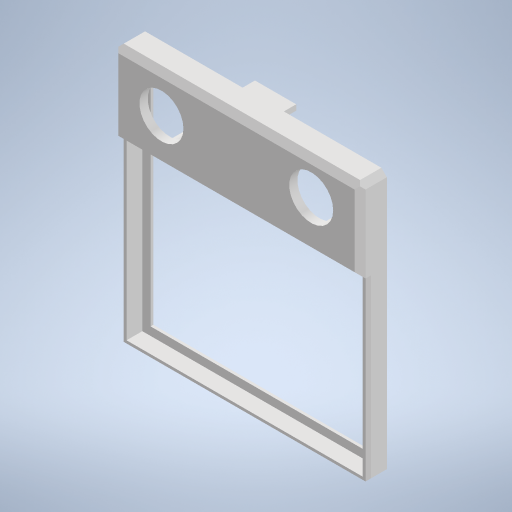
# Autodesk Inventor part: Top
Saved by Autodesk Inventor 2023.1 (Build 271208000, 208)
## iProperties
Created: 2023-03-16
Part Number: Top
Material: Generisch
Document SubType Name: Modeling
Designer: nikla
Density: 1 g/cm^3
Appearance: Vorgabe
Author: nikla
Autodesk Inventor part; units mm, degrees
ref_plane "YZ Plane" through (0, 0, 0) normal (1, 0, 0) x (0, 1, 0)
ref_plane "XZ Plane" through (0, 0, 0) normal (0, 1, 0) x (-1, 0, 0)
ref_plane "XY Plane" through (0, 0, 0) normal (0, 0, 1) x (1, 0, 0)
sketch "Skizze1" plane through (0, 0, 0) normal (0, 0, 1) x (1, 0, 0)
  line L0 (44.95, -45.95) -> (44.95, 45.95) projected
  line L1 (42.95, 47.95) -> (7.5, 47.95) projected
  line L2 (7.5, 44.95) -> (7.5, 47.95) projected
  line L3 (15, 44.95) -> (7.5, 44.95) projected
  line L4 (15, 44.95) -> (15, 42.95) projected
  line L5 (15, 42.95) -> (39.95, 42.95) projected
  line L6 (39.95, 42.95) -> (39.95, -42.95) projected
  line L7 (39.95, -42.95) -> (-39.95, -42.95) projected
  line L8 (-39.95, -42.95) -> (-39.95, 42.95) projected
  line L9 (-39.95, 42.95) -> (-15, 42.95) projected
  line L10 (-15, 42.95) -> (-15, 44.95) projected
  line L11 (-7.5, 44.95) -> (-15, 44.95) projected
  line L12 (-7.5, 47.95) -> (-7.5, 44.95) projected
  line L13 (-42.95, 47.95) -> (-7.5, 47.95) projected
  line L14 (-44.95, 45.95) -> (-44.95, -45.95) projected
  line L15 (-42.95, -47.95) -> (42.95, -47.95) projected
  line L16 (-44.95, 47.95) -> (44.95, 47.95)
  line L17 (44.95, 47.95) -> (44.95, -47.95)
  line L18 (44.95, -47.95) -> (-44.95, -47.95)
  line L19 (-44.95, -47.95) -> (-44.95, 47.95)
  line L20 (-15, 42.95) -> (-15, 36.95)
  line L21 (-15, 36.95) -> (-39.95, 36.95)
  line L22 (0, -67.13) -> (0, 67.13) projected
  line L23 (15, 42.95) -> (15, 36.95)
  line L24 (15, 36.95) -> (39.95, 36.95)
  line L25 (-39.95, -39.95) -> (-39.95, 36.95)
  line L26 (36.95, -42.95) -> (-36.95, -42.95)
  line L27 (-15, 42.95) -> (15, 42.95)
  line L28 (39.95, 36.95) -> (39.95, -39.95)
  line L29 (39.95, -39.95) -> (39.95, -42.95)
  line L30 (36.95, -42.95) -> (39.95, -42.95)
  line L31 (-36.95, -42.95) -> (-39.95, -42.95)
  line L32 (-39.95, -39.95) -> (-39.95, -42.95)
  line L33 (-44.95, 45.95) -> (-42.95, 47.95) projected
  line L34 (-42.95, -47.95) -> (-44.95, -45.95) projected
  line L35 (44.95, -45.95) -> (42.95, -47.95) projected
  line L36 (42.95, 47.95) -> (44.95, 45.95) projected
  point P0 (0, 0)
  point P1 (-15, 43.95)
  point P2 (-15, 39.95)
  constraints: 34 end point, 5 symmetric about line, 4 collinear, 4 parallel, 2 horizontal, 2 midpoint, 2 perpendicular, 1 vertical alignment
extrude "Extrusion1" add sketch "Skizze1" along normal blind 1 contours L35 L15 L22 L7 L6 L5 L4 L3 L2 L1 L36 L0 | L15 L34 L14 L33 L13 L12 L11 L10 L9 L8 L7 L22 | L20 L21 L8 L9 | L5 L6 L24 L23
sketch "Skizze2" plane through (0, 0, 1) normal (0, 0, 1) x (1, 0, 0)
  line L0 (44.95, -45.95) -> (44.95, 45.95) projected
  line L1 (-44.95, -47.95) -> (44.95, -47.95)
  line L2 (44.95, -47.95) -> (44.95, 47.95)
  line L3 (44.95, 47.95) -> (-44.95, 47.95)
  line L4 (-44.95, 47.95) -> (-44.95, -47.95)
  line L5 (-42.95, -45.95) -> (42.95, -45.95)
  line L6 (42.95, -45.95) -> (42.95, 45.95)
  line L7 (42.95, 45.95) -> (-42.95, 45.95)
  line L8 (-42.95, 45.95) -> (-42.95, -45.95)
  point P0 (0, 0)
  point P1 (44.95, -47.95)
  point P2 (44.95, -47.95)
  point P3 (44.95, -44.95)
  point P4 (44.95, 44.95)
  point P5 (44.95, -44.95)
  point P6 (44.95, 44.95)
  dimension "d5" = 2
  dimension "d6" = 2
  dimension "d7" = 2
  dimension "d8" = 2
  constraints: 16 end point, 4 parallel, 2 horizontal, 2 perpendicular
  measures "d5" distance between parallel lines of L1 L5
  measures "d6" distance between parallel lines of L3 L7
  measures "d7" distance between parallel lines of L4 L8
  measures "d8" distance between parallel lines of L0 L6
extrude "Extrusion2" add sketch "Skizze2" along normal blind 5.75
sketch "Skizze3" plane through (0, 0, 6.75) normal (0, 0, 1) x (1, 0, 0)
  line L0 (44.95, -45.95) -> (44.95, 45.95) projected
  line L1 (-44.95, 45.95) -> (-44.95, -45.95) projected
  line L2 (44.95, 47.95) -> (-44.95, 47.95)
  line L3 (-44.95, 47.95) -> (-44.95, 17.95)
  line L4 (-44.95, 17.95) -> (44.95, 17.95)
  line L5 (44.95, 17.95) -> (44.95, 47.95)
  circle A0 centre (27.1853, 35.5383) radius 1.75 projected
  circle A1 centre (-27.25, 34.028) radius 1.75 projected
  circle A2 centre (-27.25, 34.028) radius 8
  circle A3 centre (27.1853, 35.5383) radius 8
  point P0 (0, 0)
  point P1 (44.95, -47.95)
  point P2 (-44.95, 47.95)
  point P3 (-44.95, -47.95)
  point P4 (-44.95, 47.95)
  point P5 (44.95, 17.95)
  point P6 (44.95, -44.95)
  point P7 (44.95, 44.95)
  point P8 (-44.95, 44.95)
  point P9 (-44.95, -44.95)
  point P10 (-44.95, 44.95)
  point P11 (44.95, 17.95)
  dimension "d11" = 30
  dimension "d12" = 16
  dimension "d13" = 16
  constraints: 8 end point, 2 centre point, 2 coincident, 2 parallel, 1 horizontal, 1 perpendicular, 1 point on line
  measures "d11" distance of L3.end L2.end
  measures "d12" diameter of A2
  measures "d13" diameter of A3
extrude "Extrusion3" add sketch "Skizze3" along normal blind 3 contours L4 L1 L3 L2 L5 L0
fillet "Rundung2" [suppressed]
fillet "Rundung3" [suppressed]
sketch "Skizze4" plane through (0, 0, 1) normal (0, 0, -1) x (-1, 0, 0)
  line L0 (7.5, 45.95) -> (7.5, 47.95) projected
  line L1 (-7.5, 47.95) -> (7.5, 47.95) projected
  line L2 (-7.5, 47.95) -> (-7.5, 45.95) projected
  line L3 (7.5, 45.95) -> (-7.5, 45.95) projected
  line L4 (7.5, 45.95) -> (-7.5, 45.95)
  line L5 (-7.5, 45.95) -> (-7.5, 47.95)
  line L6 (-7.5, 47.95) -> (7.5, 47.95)
  line L7 (7.5, 47.95) -> (7.5, 45.95)
  point P0 (0, 0)
  constraints: 8 end point, 2 parallel, 1 horizontal, 1 perpendicular
extrude "Extrusion4" add sketch "Skizze4" along normal blind 5.5
chamfer "Fase1" distance 1 angle 45 3 edges at (-44.95, -15, 6.75) (0, -47.95, 6.75) (44.95, -15, 6.75)
sketch "Skizze5" plane through (0, 0, 6.75) normal (0, 0, -1) x (-1, 0, 0)
  circle A0 centre (26.75, 21.7) radius 1.1 projected
  circle A1 centre (-27.25, 21.65) radius 1.1 projected
  circle A2 centre (26.75, 21.7) radius 2.75
  circle A3 centre (-27.25, 21.65) radius 2.75
  circle A4 centre (26.75, 21.7) radius 0.9
  circle A5 centre (-27.25, 21.65) radius 0.9
  point P0 (0, 0)
  dimension "d24" = 5.5
  dimension "d25" = 5.5
  dimension "d26" = 1.8
  dimension "d27" = 1.8
  constraints: 4 centre point, 4 coincident
  measures "d24" diameter of A2
  measures "d25" diameter of A3
  measures "d26" diameter of A4
  measures "d27" diameter of A5
extrude "Extrusion5" add sketch "Skizze5" along normal blind 6.5 contours A0 | A1 | A2 | A3
chamfer "Fase2" distance 2 angle 45 4 edges at (-44.95, 32.95, 9.75) (0, 47.95, 9.75) (0, 17.95, 9.75) (44.95, 32.95, 9.75)
chamfer "Fase3" distance 2 angle 45 4 edges at (-44.95, -47.95, 3.375) (-44.95, 47.95, 4.375) (44.95, -47.95, 3.375) (44.95, 47.95, 4.375)
